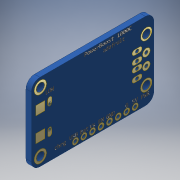
# Autodesk Inventor part: PlacaSuperboost1000C
Saved by Autodesk Inventor 2018 (Build 220112000, 112)
## iProperties
Created: 2018-01-30
Part Number: PlacaSuperboost1000C
Material: Genérico
Document SubType Name: Modeling
Designer: RafaX
Density: 1 g/cm^3
Appearance: Valor por defecto
Author: RafaX
Autodesk Inventor part; units mm, degrees
(part 1 of 2)
ref_plane "YZ Plane" through (0, 0, 0) normal (1, 0, 0) x (0, 1, 0)
ref_plane "XZ Plane" through (0, 0, 0) normal (0, 1, 0) x (-1, 0, 0)
ref_plane "PlanoCurre" through (0, 0, 0) normal (0, -1, 0) x (1, 0, 0)
sketch "FOTO_PLANO" plane through (0, 0, 0) normal (0, -1, 0) x (1, 0, 0)
  line L0 (-28.5613, 4.3764) -> (30.0496, 4.3764)
  line L1 (30.0496, 4.3764) -> (30.0496, -40.7266)
  line L2 (30.0496, -40.7266) -> (-28.5613, -40.7266)
  line L3 (-28.5613, -40.7266) -> (-28.5613, 4.3764)
  point P0 (0, 0)
  constraints: 2 other
sketch "BocetoPCB" plane through (0, 0, 0) normal (0, -1, 0) x (1, 0, 0)
  line L0 (-20.36, 0) -> (-2.5, 0)
  line L1 (0, -2.5) -> (0, -33.7)
  line L2 (-2.5, -36.2) -> (-20.36, -36.2)
  line L3 (-22.86, -33.7) -> (-22.86, -2.5)
  arc A0 (-20.36, 0) -> (-22.86, -2.5) centre (-20.36, -2.5) ccw
  arc A1 (0, -2.5) -> (-2.5, 0) centre (-2.5, -2.5) ccw
  arc A2 (-2.5, -36.2) -> (0, -33.7) centre (-2.5, -33.7) ccw
  arc A3 (-22.86, -33.7) -> (-20.36, -36.2) centre (-20.36, -33.7) ccw
  point P0 (-22.86, 0)
  point P1 (0, -36.2)
  point P2 (0, 0)
  point P3 (-20.255, -2.6419)
  point P4 (-2.605, -2.6419)
  point P5 (-0.0135, -33.9591)
  point P6 (-18.2509, -33.9512)
  point P7 (-5.1628, -33.9437)
  constraints: 9 point on circle, 8 end point, 8 tangent, 6 point on line, 4 centre point, 2 equal radius, 2 parallel, 1 horizontal, 1 perpendicular
extrude "board" add sketch "BocetoPCB" along normal blind 1.588
hole "Agujeros" at (-20.255, 0, -2.6419) at (-2.605, 0, -2.6419) at (-18.2509, 0, -33.9512) at (-5.1628, 0, -33.9437) direction (0, -1, 0) diameter 2.4 end through all
sketch "Boceto4" plane through (0, 0, 0) normal (0, 1, 0) x (1, 0, 0)
  circle A0 centre (-2.6033, 2.6414) radius 1.7995
  circle A1 centre (-2.6033, 2.6414) radius 1.2026
  circle A2 centre (-20.2425, 2.6414) radius 1.2088
  circle A3 centre (-20.2425, 2.6414) radius 1.8114
  circle A4 centre (-1.259, 13.0031) radius 0.4663
  circle A5 centre (-1.259, 13.0031) radius 0.9026
  circle A6 centre (-1.259, 15.5106) radius 0.4663
  circle A7 centre (-1.259, 15.5106) radius 0.9026
  circle A8 centre (-1.259, 18.0275) radius 0.4663
  circle A9 centre (-1.259, 18.0275) radius 0.9026
  circle A10 centre (-1.259, 20.5673) radius 0.4663
  circle A11 centre (-1.259, 20.5673) radius 0.9026
  circle A12 centre (-1.259, 23.0791) radius 0.4663
  circle A13 centre (-1.259, 23.0791) radius 0.9026
  circle A14 centre (-1.259, 25.6387) radius 0.4663
  circle A15 centre (-1.259, 25.6387) radius 0.9026
  circle A16 centre (-1.259, 28.1385) radius 0.4663
  circle A17 centre (-1.259, 28.1385) radius 0.9026
  circle A18 centre (-1.259, 30.6623) radius 0.4663
  circle A19 centre (-1.259, 30.6623) radius 0.9026
  circle A20 centre (-18.2509, 33.9512) radius 1.2 projected
  circle A21 centre (-18.2509, 33.9512) radius 1.2
  circle A22 centre (-18.2509, 33.9512) radius 1.6562
  circle A23 centre (-5.1628, 33.9437) radius 1.2 projected
  circle A24 centre (-5.1628, 33.9437) radius 1.2
  circle A25 centre (-5.1628, 33.9437) radius 1.6796
  circle A26 centre (-8.2006, 31.2204) radius 0.476
  line L0 (-8.2006, 29.7597) -> (-8.2006, 32.6808) construction
  line L1 (-7.4792, 30.4811) -> (-7.4792, 31.9594)
  line L2 (-8.9221, 31.9594) -> (-8.9221, 30.4811)
  arc A27 (-8.9221, 30.4811) -> (-7.4792, 30.4811) centre (-8.2006, 30.4811) ccw
  arc A28 (-7.4792, 31.9594) -> (-8.9221, 31.9594) centre (-8.2006, 31.9594) ccw
  circle A29 centre (-10.7403, 31.2204) radius 0.476
  line L3 (-10.0189, 30.4811) -> (-10.0189, 31.9594)
  line L4 (-11.4617, 31.9594) -> (-11.4617, 30.4811)
  arc A30 (-11.4617, 30.4811) -> (-10.0189, 30.4811) centre (-10.7403, 30.4811) ccw
  arc A31 (-10.0189, 31.9594) -> (-11.4617, 31.9594) centre (-10.7403, 31.9594) ccw
  circle A32 centre (-12.6758, 31.2204) radius 0.476
  line L5 (-11.9544, 30.4811) -> (-11.9544, 31.9594)
  line L6 (-13.3972, 31.9594) -> (-13.3972, 30.4811)
  arc A33 (-13.3972, 30.4811) -> (-11.9544, 30.4811) centre (-12.6758, 30.4811) ccw
  arc A34 (-11.9544, 31.9594) -> (-13.3972, 31.9594) centre (-12.6758, 31.9594) ccw
  circle A35 centre (-15.2037, 31.2204) radius 0.476
  line L7 (-14.4823, 30.4811) -> (-14.4823, 31.9594)
  line L8 (-15.9251, 31.9594) -> (-15.9251, 30.4811)
  arc A36 (-15.9251, 30.4811) -> (-14.4823, 30.4811) centre (-15.2037, 30.4811) ccw
  arc A37 (-14.4823, 31.9594) -> (-15.9251, 31.9594) centre (-15.2037, 31.9594) ccw
  line L9 (-16.2221, 1.3283) -> (-13.5843, 1.3283)
  line L10 (-13.5843, 1.3283) -> (-13.5843, 3.9523)
  line L11 (-13.5843, 3.9523) -> (-16.2221, 3.9523)
  line L12 (-16.2221, 3.9523) -> (-16.2221, 1.3283)
  line L13 (-9.0492, 1.3283) -> (-6.4567, 1.3283)
  line L14 (-6.4567, 1.3283) -> (-6.4567, 3.9523)
  line L15 (-6.4567, 3.9523) -> (-9.0492, 3.9523)
  line L16 (-9.0492, 3.9523) -> (-9.0492, 1.3283)
  line L17 (-16.4659, 5.4151) -> (-14.0753, 5.4151) construction
  line L18 (-15.8504, 4.7996) -> (-14.6908, 4.7996)
  line L19 (-14.6908, 6.0305) -> (-15.8504, 6.0305)
  arc A38 (-15.8504, 6.0305) -> (-15.8504, 4.7996) centre (-15.8504, 5.4151) ccw
  arc A39 (-14.6908, 4.7996) -> (-14.6908, 6.0305) centre (-14.6908, 5.4151) ccw
  circle A40 centre (-14.6284, 5.4151) radius 0.2973
  line L20 (-8.7027, 5.4177) -> (-6.2957, 5.4177) construction
  line L21 (-8.1043, 4.8193) -> (-6.8941, 4.8193)
  line L22 (-6.8941, 6.0161) -> (-8.1043, 6.0161)
  arc A41 (-8.1043, 6.0161) -> (-8.1043, 4.8193) centre (-8.1043, 5.4177) ccw
  arc A42 (-6.8941, 4.8193) -> (-6.8941, 6.0161) centre (-6.8941, 5.4177) ccw
  circle A43 centre (-8.1673, 5.4177) radius 0.2995
  circle A44 centre (-3.4049, 35.326) radius 0.1393
  circle A45 centre (-3.4049, 35.326) radius 0.4359
  circle A46 centre (-10.0649, 33.9437) radius 0.4442
  circle A47 centre (-10.0649, 33.9437) radius 1.1154
  circle A48 centre (-13.5064, 33.9548) radius 0.4442
  circle A49 centre (-13.5064, 33.9548) radius 1.1154
  line L23 (0, 33.7) -> (0, 2.5) projected
  circle A50 centre (-18.2509, 33.9512) radius 1.2 projected
  circle A51 centre (-20.255, 2.6419) radius 1.2 projected
  circle A52 centre (-2.605, 2.6419) radius 1.2 projected
  circle A53 centre (-5.1628, 33.9437) radius 1.2 projected
  line L24 (0, 2.5) -> (0, 33.7) projected
  arc A54 (0, 33.7) -> (-2.5, 36.2) centre (-2.5, 33.7) ccw projected
  line L25 (-2.5, 36.2) -> (-20.36, 36.2) projected
  arc A55 (-20.36, 36.2) -> (-22.86, 33.7) centre (-20.36, 33.7) ccw projected
  line L26 (-22.86, 33.7) -> (-22.86, 2.5) projected
  arc A56 (-22.86, 2.5) -> (-20.36, 0) centre (-20.36, 2.5) ccw projected
  line L27 (-20.36, 0) -> (-2.5, 0) projected
  arc A57 (-2.5, 0) -> (0, 2.5) centre (-2.5, 2.5) ccw projected
  point P0 (0, 0)
  point P1 (-8.2006, 31.2203)
  point P2 (-15.2706, 5.4151)
  point P3 (-7.4992, 5.4177)
  point P4 (-8.2006, 31.2203)
  constraints: 52 end point, 48 centre point, 30 point on circle, 24 tangent, 18 coincident, 10 parallel, 10 point on line, 4 horizontal, 3 midpoint, 2 perpendicular, 1 vertical
extrude "Extrusión3" add sketch "Boceto4" along normal blind 0.02 separate body contours A0 | A3 | A5 | A7 | A9 | A11 | A13 | A15 | A17 | A19 | A22 | A25 | A27 L2 A28 L1 | A30 L4 A31 L3 | A33 L6 A34 L5 | A36 L8 A37 L7 | L12 L11 L10 L9 | L16 L15 L14 L13 | A38 L19 A39 L18 | A41 L22 A42 L21 | A47 | A49
hole "Agujero4" at (-13.5064, 0, -33.9548) direction (0, -1, 0) diameter 1 end through all bodies 1
hole "Agujero5" at (-13.5064, 0, -33.9548) at (-10.0649, 0, -33.9437) at (-10.7403, 0, -31.2204) at (-12.6758, 0, -31.2204) at (-15.2037, 0, -31.2204) at (-8.2006, 0, -31.2203) at (-1.259, 0, -25.6387) at (-1.259, 0, -28.1385) at (-1.259, 0, -30.6623) at (-1.259, 0, -23.0791) at (-1.259, 0, -20.5673) at (-1.259, 0, -18.0275) at (-1.259, 0, -15.5106) at (-1.259, 0, -13.0031) at (-8.1673, 0, -5.4177) at (-14.6284, 0, -5.4151) direction (0, -1, 0) diameter 1 end through all bodies 1
sketch "textos" plane through (0, 0, 0) normal (0, 1, 0) x (1, 0, 0)
  line L0 (-22.5433, 15.6124) -> (-22.5433, 35.6124) construction
  line L1 (-22.5433, 35.6124) -> (-20.8728, 35.6124) construction
  line L2 (-20.8728, 35.6124) -> (-20.8728, 15.6124) construction
  line L3 (-20.8728, 15.6124) -> (-22.5433, 15.6124) construction
  line L4 (-20.9084, 21.173) -> (-20.9084, 28.7586) construction
  line L5 (-20.9084, 28.7586) -> (-19.6941, 28.7586) construction
  line L6 (-19.6941, 28.7586) -> (-19.6941, 21.173) construction
  line L7 (-19.6941, 21.173) -> (-20.9084, 21.173) construction
  line L8 (-3.3208, 11.209) -> (-3.3208, 13.795) construction
  line L9 (-3.3208, 13.795) -> (-2.293, 13.795) construction
  line L10 (-2.293, 13.795) -> (-2.293, 11.209) construction
  line L11 (-2.293, 11.209) -> (-3.3208, 11.209) construction
  line L12 (-3.274, 14.3294) -> (-3.274, 17.056) construction
  line L13 (-3.274, 17.056) -> (-2.274, 17.056) construction
  line L14 (-2.274, 17.056) -> (-2.274, 14.3294) construction
  line L15 (-2.274, 14.3294) -> (-3.274, 14.3294) construction
  line L16 (-3.2305, 17.2189) -> (-3.2305, 18.9429) construction
  line L17 (-3.2305, 18.9429) -> (-2.2171, 18.9429) construction
  line L18 (-2.2171, 18.9429) -> (-2.2171, 17.2189) construction
  line L19 (-2.2171, 17.2189) -> (-3.2305, 17.2189) construction
  line L20 (-3.274, 19.6989) -> (-3.274, 21.4229) construction
  line L21 (-3.274, 21.4229) -> (-2.274, 21.4229) construction
  line L22 (-2.274, 21.4229) -> (-2.274, 19.6989) construction
  line L23 (-2.274, 19.6989) -> (-3.274, 19.6989) construction
  line L24 (-3.3018, 22.0618) -> (-3.3018, 24.6478) construction
  line L25 (-3.3018, 24.6478) -> (-2.274, 24.6478) construction
  line L26 (-2.274, 24.6478) -> (-2.274, 22.0618) construction
  line L27 (-2.274, 22.0618) -> (-3.3018, 22.0618) construction
  line L28 (-3.3777, 27.7538) -> (-3.3777, 28.6158) construction
  line L29 (-3.3777, 28.6158) -> (-2.3499, 28.6158) construction
  line L30 (-2.3499, 28.6158) -> (-2.3499, 27.7538) construction
  line L31 (-2.3499, 27.7538) -> (-3.3777, 27.7538) construction
  line L32 (-3.3823, 29.7413) -> (-3.3823, 31.4654) construction
  line L33 (-3.3823, 31.4654) -> (-2.3689, 31.4654) construction
  line L34 (-2.3689, 31.4654) -> (-2.3689, 29.7413) construction
  line L35 (-2.3689, 29.7413) -> (-3.3823, 29.7413) construction
  line L36 (-3.255, 32.3541) -> (-3.255, 34.9402) construction
  line L37 (-3.255, 34.9402) -> (-2.255, 34.9402) construction
  line L38 (-2.255, 34.9402) -> (-2.255, 32.3541) construction
  line L39 (-2.255, 32.3541) -> (-3.255, 32.3541) construction
  line L40 (-3.0732, 6.7716) -> (-3.0732, 10.2196) construction
  line L41 (-3.0732, 10.2196) -> (-1.6699, 10.2196) construction
  line L42 (-1.6699, 10.2196) -> (-1.6699, 6.7716) construction
  line L43 (-1.6699, 6.7716) -> (-3.0732, 6.7716) construction
  line L44 (-18.5708, 4.0743) -> (-18.5708, 6.6604) construction
  line L45 (-18.5708, 6.6604) -> (-17.5431, 6.6604) construction
  line L46 (-17.5431, 6.6604) -> (-17.5431, 4.0743) construction
  line L47 (-17.5431, 4.0743) -> (-18.5708, 4.0743) construction
  line L48 (-17.5565, 4.8279) -> (-17.5565, 4.2527)
  line L49 (-17.5565, 4.2527) -> (-18.5565, 4.2527)
  line L50 (-18.5565, 4.2527) -> (-18.5565, 4.3915)
  line L51 (-18.5565, 4.3915) -> (-17.673, 4.3915)
  line L52 (-17.673, 4.3915) -> (-17.673, 4.8279)
  line L53 (-17.673, 4.8279) -> (-17.5565, 4.8279)
  spline S0 degree 2 poles (-18.0637, 5.7562) (-17.9284, 5.7562) (-17.733, 5.6926) (-17.6049, 5.5851) (-17.5431, 5.4399) (-17.5431, 5.3602) knots 0 0 0 1 2 3 4 4 4
  spline S1 degree 2 poles (-17.5431, 5.3602) (-17.5431, 5.2634) (-17.613, 5.12) (-17.7447, 5.026) (-17.9337, 4.9803) (-18.052, 4.9803) knots 0 0 0 1 2 3 4 4 4
  spline S2 degree 2 poles (-18.052, 4.9803) (-18.1855, 4.9803) (-18.3809, 5.043) (-18.509, 5.1505) (-18.5708, 5.2948) (-18.5708, 5.3754) knots 0 0 0 1 2 3 4 4 4
  spline S3 degree 2 poles (-18.5708, 5.3754) (-18.5708, 5.4713) (-18.5001, 5.6147) (-18.3692, 5.7096) (-18.1811, 5.7562) (-18.0637, 5.7562) knots 0 0 0 1 2 3 4 4 4
  spline S4 degree 2 poles (-18.0538, 5.62) (-18.1416, 5.62) (-18.2877, 5.5923) (-18.3934, 5.5313) (-18.4517, 5.4355) (-18.4517, 5.3674) knots 0 0 0 1 2 3 4 4 4
  spline S5 degree 2 poles (-18.4517, 5.3674) (-18.4517, 5.3019) (-18.3898, 5.207) (-18.2832, 5.146) (-18.1398, 5.1165) (-18.0592, 5.1165) knots 0 0 0 1 2 3 4 4 4
  spline S6 degree 2 poles (-18.0592, 5.1165) (-17.9705, 5.1165) (-17.8244, 5.1442) (-17.7196, 5.2052) (-17.6613, 5.3002) (-17.6613, 5.3674) knots 0 0 0 1 2 3 4 4 4
  spline S7 degree 2 poles (-17.6613, 5.3674) (-17.6613, 5.4328) (-17.7232, 5.5286) (-17.8298, 5.5905) (-17.9723, 5.62) (-18.0538, 5.62) knots 0 0 0 1 2 3 4 4 4
  line L54 (-18.5565, 6.6254) -> (-17.5565, 6.5582)
  line L55 (-17.5565, 6.5582) -> (-17.5565, 6.3817)
  line L56 (-17.5565, 6.3817) -> (-17.9122, 6.2571)
  line L57 (-17.9122, 6.2571) -> (-18.026, 6.2231)
  line L58 (-18.026, 6.2231) -> (-17.9033, 6.1872)
  line L59 (-17.9033, 6.1872) -> (-17.5565, 6.0717)
  line L60 (-17.5565, 6.0717) -> (-17.5565, 5.9014)
  line L61 (-17.5565, 5.9014) -> (-18.5565, 5.8324)
  line L62 (-18.5565, 5.8324) -> (-18.5565, 5.9605)
  line L63 (-18.5565, 5.9605) -> (-17.8755, 6)
  line L64 (-17.8755, 6) -> (-17.6891, 6.0116)
  line L65 (-17.6891, 6.0116) -> (-17.8477, 6.06)
  line L66 (-17.8477, 6.06) -> (-18.2187, 6.181)
  line L67 (-18.2187, 6.181) -> (-18.2187, 6.2751)
  line L68 (-18.2187, 6.2751) -> (-17.8208, 6.4148)
  line L69 (-17.8208, 6.4148) -> (-17.6891, 6.4614)
  line L70 (-17.6891, 6.4614) -> (-17.8262, 6.4641)
  line L71 (-17.8262, 6.4641) -> (-18.5565, 6.5036)
  line L72 (-18.5565, 6.5036) -> (-18.5565, 6.6254)
  line L73 (-19.8179, 21.7456) -> (-19.9209, 21.7429)
  spline S8 degree 2 poles (-19.9209, 21.7429) (-19.8591, 21.6846) (-19.8045, 21.5646) (-19.8045, 21.4983) knots 0 0 0 1 2 2 2
  spline S9 degree 2 poles (-19.8045, 21.4983) (-19.8045, 21.4373) (-19.8376, 21.3504) (-19.8968, 21.294) (-19.9765, 21.268) (-20.0231, 21.268) knots 0 0 0 1 2 3 4 4 4
  spline S10 degree 2 poles (-20.0231, 21.268) (-20.1387, 21.268) (-20.2695, 21.4275) (-20.2695, 21.5843) knots 0 0 0 1 2 2 2
  line L74 (-20.2695, 21.5843) -> (-20.2695, 21.7321)
  line L75 (-20.2695, 21.7321) -> (-20.3367, 21.7321)
  spline S11 degree 2 poles (-20.3367, 21.7321) (-20.4048, 21.7321) (-20.4864, 21.6515) (-20.4864, 21.5681) knots 0 0 0 1 2 2 2
  spline S12 degree 2 poles (-20.4864, 21.5681) (-20.4864, 21.5072) (-20.4577, 21.3898) (-20.4308, 21.3271) knots 0 0 0 1 2 2 2
  line L76 (-20.4308, 21.3271) -> (-20.5509, 21.3271)
  spline S13 degree 2 poles (-20.5509, 21.3271) (-20.5598, 21.3504) (-20.5778, 21.4086) (-20.5912, 21.4723) (-20.6002, 21.5422) (-20.6002, 21.578) knots 0 0 0 1 2 3 4 4 4
  spline S14 degree 2 poles (-20.6002, 21.578) (-20.6002, 21.6425) (-20.5697, 21.7465) (-20.507, 21.8181) (-20.412, 21.8567) (-20.3475, 21.8567) knots 0 0 0 1 2 3 4 4 4
  line L77 (-20.3475, 21.8567) -> (-19.8179, 21.8567)
  line L78 (-19.8179, 21.8567) -> (-19.8179, 21.7456)
  line L79 (-20.1674, 21.7321) -> (-20.1674, 21.5753)
  spline S15 degree 2 poles (-20.1674, 21.5753) (-20.1674, 21.5287) (-20.1476, 21.4615) (-20.1109, 21.4194) (-20.0598, 21.3988) (-20.0276, 21.3988) knots 0 0 0 1 2 3 4 4 4
  spline S16 degree 2 poles (-20.0276, 21.3988) (-20.0052, 21.3988) (-19.9649, 21.4113) (-19.9335, 21.44) (-19.9147, 21.4857) (-19.9147, 21.518) knots 0 0 0 1 2 3 4 4 4
  spline S17 degree 2 poles (-19.9147, 21.518) (-19.9147, 21.561) (-19.9711, 21.6712) (-20.0312, 21.7321) knots 0 0 0 1 2 2 2
  line L80 (-20.0312, 21.7321) -> (-20.1674, 21.7321)
  spline S18 degree 2 poles (-20.1862, 22.052) (-20.2838, 22.052) (-20.4362, 22.1013) (-20.541, 22.1936) (-20.5957, 22.3217) (-20.5957, 22.4006) knots 0 0 0 1 2 3 4 4 4
  spline S19 degree 2 poles (-20.5957, 22.4006) (-20.5957, 22.4346) (-20.5858, 22.5009) (-20.576, 22.5332) knots 0 0 0 1 2 2 2
  line L81 (-20.576, 22.5332) -> (-20.8994, 22.5332)
  line L82 (-20.8994, 22.5332) -> (-20.8994, 22.6577)
  line L83 (-20.8994, 22.6577) -> (-19.8179, 22.6577)
  line L84 (-19.8179, 22.6577) -> (-19.8179, 22.5466)
  line L85 (-19.8179, 22.5466) -> (-19.9631, 22.5422)
  spline S20 degree 2 poles (-19.9631, 22.5422) (-19.8824, 22.4902) (-19.8045, 22.3692) (-19.8045, 22.2993) knots 0 0 0 1 2 2 2
  spline S21 degree 2 poles (-19.8045, 22.2993) (-19.8045, 22.2384) (-19.8591, 22.1452) (-19.9595, 22.0825) (-20.1002, 22.052) (-20.1862, 22.052) knots 0 0 0 1 2 3 4 4 4
  spline S22 degree 2 poles (-20.1942, 22.1784) (-20.0554, 22.1784) (-19.9183, 22.2545) (-19.9183, 22.3244) knots 0 0 0 1 2 2 2
  spline S23 degree 2 poles (-19.9183, 22.3244) (-19.9183, 22.371) (-20.0088, 22.4758) (-20.0975, 22.5332) knots 0 0 0 1 2 2 2
  line L86 (-20.0975, 22.5332) -> (-20.4541, 22.5332)
  spline S24 degree 2 poles (-20.4541, 22.5332) (-20.4693, 22.5027) (-20.4855, 22.4284) (-20.4855, 22.3925) knots 0 0 0 1 2 2 2
  spline S25 degree 2 poles (-20.4855, 22.3925) (-20.4855, 22.2913) (-20.3448, 22.1784) (-20.1942, 22.1784) knots 0 0 0 1 2 2 2
  line L87 (-19.8179, 23.3477) -> (-19.9209, 23.345)
  spline S26 degree 2 poles (-19.9209, 23.345) (-19.8591, 23.2868) (-19.8045, 23.1667) (-19.8045, 23.1004) knots 0 0 0 1 2 2 2
  spline S27 degree 2 poles (-19.8045, 23.1004) (-19.8045, 23.0395) (-19.8376, 22.9526) (-19.8968, 22.8961) (-19.9765, 22.8701) (-20.0231, 22.8701) knots 0 0 0 1 2 3 4 4 4
  spline S28 degree 2 poles (-20.0231, 22.8701) (-20.1387, 22.8701) (-20.2695, 23.0296) (-20.2695, 23.1864) knots 0 0 0 1 2 2 2
  line L88 (-20.2695, 23.1864) -> (-20.2695, 23.3343)
  line L89 (-20.2695, 23.3343) -> (-20.3367, 23.3343)
  spline S29 degree 2 poles (-20.3367, 23.3343) (-20.4048, 23.3343) (-20.4864, 23.2536) (-20.4864, 23.1703) knots 0 0 0 1 2 2 2
  spline S30 degree 2 poles (-20.4864, 23.1703) (-20.4864, 23.1094) (-20.4577, 22.992) (-20.4308, 22.9293) knots 0 0 0 1 2 2 2
  line L90 (-20.4308, 22.9293) -> (-20.5509, 22.9293)
  spline S31 degree 2 poles (-20.5509, 22.9293) (-20.5598, 22.9526) (-20.5778, 23.0108) (-20.5912, 23.0744) (-20.6002, 23.1443) (-20.6002, 23.1802) knots 0 0 0 1 2 3 4 4 4
  spline S32 degree 2 poles (-20.6002, 23.1802) (-20.6002, 23.2447) (-20.5697, 23.3486) (-20.507, 23.4203) (-20.412, 23.4588) (-20.3475, 23.4588) knots 0 0 0 1 2 3 4 4 4
  line L91 (-20.3475, 23.4588) -> (-19.8179, 23.4588)
  line L92 (-19.8179, 23.4588) -> (-19.8179, 23.3477)
  line L93 (-20.1674, 23.3343) -> (-20.1674, 23.1775)
  spline S33 degree 2 poles (-20.1674, 23.1775) (-20.1674, 23.1309) (-20.1476, 23.0637) (-20.1109, 23.0215) (-20.0598, 23.0009) (-20.0276, 23.0009) knots 0 0 0 1 2 3 4 4 4
  spline S34 degree 2 poles (-20.0276, 23.0009) (-20.0052, 23.0009) (-19.9649, 23.0135) (-19.9335, 23.0422) (-19.9147, 23.0879) (-19.9147, 23.1201) knots 0 0 0 1 2 3 4 4 4
  spline S35 degree 2 poles (-19.9147, 23.1201) (-19.9147, 23.1631) (-19.9711, 23.2733) (-20.0312, 23.3343) knots 0 0 0 1 2 2 2
  line L94 (-20.0312, 23.3343) -> (-20.1674, 23.3343)
  spline S36 degree 2 poles (-20.7749, 24.3235) (-20.7973, 24.2267) (-20.7973, 24.156) knots 0 0 0 1 1 1
  spline S37 degree 2 poles (-20.7973, 24.156) (-20.7973, 23.9884) (-20.6091, 23.9884) knots 0 0 0 1 1 1
  line L95 (-20.6091, 23.9884) -> (-20.4747, 23.9884)
  line L96 (-20.4747, 23.9884) -> (-20.4747, 24.302)
  line L97 (-20.4747, 24.302) -> (-20.3636, 24.302)
  line L98 (-20.3636, 24.302) -> (-20.3636, 23.9884)
  line L99 (-20.3636, 23.9884) -> (-19.8179, 23.9884)
  line L100 (-19.8179, 23.9884) -> (-19.8179, 23.8629)
  line L101 (-19.8179, 23.8629) -> (-20.3636, 23.8629)
  line L102 (-20.3636, 23.8629) -> (-20.3636, 23.6336)
  line L103 (-20.3636, 23.6336) -> (-20.4747, 23.6336)
  line L104 (-20.4747, 23.6336) -> (-20.4747, 23.8629)
  line L105 (-20.4747, 23.8629) -> (-20.602, 23.8629)
  spline S38 degree 2 poles (-20.602, 23.8629) (-20.9084, 23.8629) (-20.9084, 24.1604) knots 0 0 0 1 1 1
  spline S39 degree 2 poles (-20.9084, 24.1604) (-20.9084, 24.2339) (-20.8896, 24.3235) knots 0 0 0 1 1 1
  line L106 (-20.8896, 24.3235) -> (-20.7749, 24.3235)
  line L107 (-20.5858, 24.5207) -> (-20.5858, 24.6336)
  line L108 (-20.5858, 24.6336) -> (-20.4442, 24.6371)
  spline S40 degree 2 poles (-20.4442, 24.6371) (-20.5267, 24.6999) (-20.6002, 24.8235) (-20.6002, 24.8862) knots 0 0 0 1 2 2 2
  spline S41 degree 2 poles (-20.6002, 24.8862) (-20.6002, 24.9974) (-20.4451, 25.1112) (-20.2928, 25.1076) knots 0 0 0 1 2 2 2
  line L109 (-20.2928, 25.1076) -> (-20.2928, 24.9821)
  spline S42 degree 2 poles (-20.2928, 24.9821) (-20.3941, 24.9839) (-20.4855, 24.9248) (-20.4855, 24.8683) knots 0 0 0 1 2 2 2
  spline S43 degree 2 poles (-20.4855, 24.8683) (-20.4855, 24.8432) (-20.4657, 24.7931) (-20.4236, 24.7393) (-20.3582, 24.6793) (-20.3116, 24.6452) knots 0 0 0 1 2 3 4 4 4
  line L110 (-20.3116, 24.6452) -> (-19.8179, 24.6452)
  line L111 (-19.8179, 24.6452) -> (-19.8179, 24.5207)
  line L112 (-19.8179, 24.5207) -> (-20.5858, 24.5207)
  line L113 (-19.8179, 25.8665) -> (-19.8179, 25.7554)
  line L114 (-19.8179, 25.7554) -> (-19.9416, 25.7509)
  spline S44 degree 2 poles (-19.9416, 25.7509) (-19.9021, 25.7187) (-19.8493, 25.6613) (-19.817, 25.6049) (-19.8045, 25.5466) (-19.8045, 25.5153) knots 0 0 0 1 2 3 4 4 4
  spline S45 degree 2 poles (-19.8045, 25.5153) (-19.8045, 25.4042) (-19.9433, 25.2922) (-20.084, 25.2922) knots 0 0 0 1 2 2 2
  line L115 (-20.084, 25.2922) -> (-20.5858, 25.2922)
  line L116 (-20.5858, 25.2922) -> (-20.5858, 25.4158)
  line L117 (-20.5858, 25.4158) -> (-20.0948, 25.4158)
  spline S46 degree 2 poles (-20.0948, 25.4158) (-19.9183, 25.4158) (-19.9183, 25.5395) knots 0 0 0 1 1 1
  spline S47 degree 2 poles (-19.9183, 25.5395) (-19.9183, 25.5628) (-19.9326, 25.6058) (-19.9684, 25.6533) (-20.0303, 25.7079) (-20.0769, 25.7429) knots 0 0 0 1 2 3 4 4 4
  line L118 (-20.0769, 25.7429) -> (-20.5858, 25.7429)
  line L119 (-20.5858, 25.7429) -> (-20.5858, 25.8665)
  line L120 (-20.5858, 25.8665) -> (-19.8179, 25.8665)
  line L121 (-20.4756, 26.337) -> (-20.4756, 26.1255)
  line L122 (-20.4756, 26.1255) -> (-20.5858, 26.1255)
  line L123 (-20.5858, 26.1255) -> (-20.5858, 26.4615)
  line L124 (-20.5858, 26.4615) -> (-19.929, 26.4615)
  line L125 (-19.929, 26.4615) -> (-19.929, 26.6748)
  line L126 (-19.929, 26.6748) -> (-19.8179, 26.6748)
  line L127 (-19.8179, 26.6748) -> (-19.8179, 26.1022)
  line L128 (-19.8179, 26.1022) -> (-19.929, 26.1022)
  line L129 (-19.929, 26.1022) -> (-19.929, 26.337)
  line L130 (-19.929, 26.337) -> (-20.4756, 26.337)
  spline S48 degree 2 poles (-20.9084, 26.38) (-20.9084, 26.4006) (-20.8923, 26.4364) (-20.8636, 26.4624) (-20.826, 26.4776) (-20.8036, 26.4776) knots 0 0 0 1 2 3 4 4 4
  spline S49 degree 2 poles (-20.8036, 26.4776) (-20.7821, 26.4776) (-20.7435, 26.4624) (-20.7149, 26.4364) (-20.6987, 26.4006) (-20.6987, 26.38) knots 0 0 0 1 2 3 4 4 4
  spline S50 degree 2 poles (-20.6987, 26.38) (-20.6987, 26.3594) (-20.7149, 26.3235) (-20.7435, 26.2975) (-20.7821, 26.2823) (-20.8036, 26.2823) knots 0 0 0 1 2 3 4 4 4
  spline S51 degree 2 poles (-20.8036, 26.2823) (-20.826, 26.2823) (-20.8636, 26.2975) (-20.8923, 26.3235) (-20.9084, 26.3594) (-20.9084, 26.38) knots 0 0 0 1 2 3 4 4 4
  spline S52 degree 2 poles (-19.8287, 27.4696) (-19.817, 27.4275) (-19.8071, 27.3379) (-19.8071, 27.2922) knots 0 0 0 1 2 2 2
  spline S53 degree 2 poles (-19.8071, 27.2922) (-19.8071, 27.1577) (-19.938, 27.0251) (-20.0733, 27.0251) knots 0 0 0 1 2 2 2
  line L131 (-20.0733, 27.0251) -> (-20.4747, 27.0251)
  line L132 (-20.4747, 27.0251) -> (-20.4747, 26.8253)
  line L133 (-20.4747, 26.8253) -> (-20.5858, 26.8253)
  line L134 (-20.5858, 26.8253) -> (-20.5858, 27.0251)
  line L135 (-20.5858, 27.0251) -> (-20.7973, 27.0251)
  line L136 (-20.7973, 27.0251) -> (-20.8322, 27.1488)
  line L137 (-20.8322, 27.1488) -> (-20.5858, 27.1488)
  line L138 (-20.5858, 27.1488) -> (-20.5858, 27.4696)
  line L139 (-20.5858, 27.4696) -> (-20.4747, 27.4696)
  line L140 (-20.4747, 27.4696) -> (-20.4747, 27.1488)
  line L141 (-20.4747, 27.1488) -> (-20.084, 27.1488)
  spline S54 degree 2 poles (-20.084, 27.1488) (-20.0016, 27.1488) (-19.9201, 27.2312) (-19.9201, 27.3101) knots 0 0 0 1 2 2 2
  spline S55 degree 2 poles (-19.9201, 27.3101) (-19.9201, 27.345) (-19.9308, 27.4257) (-19.9433, 27.4696) knots 0 0 0 1 2 2 2
  line L142 (-19.9433, 27.4696) -> (-19.8287, 27.4696)
  spline S56 degree 2 poles (-22.1992, 16.426) (-22.1212, 16.426) (-21.9886, 16.3722) (-21.8918, 16.2683) (-21.839, 16.1124) (-21.839, 16.0093) knots 0 0 0 1 2 3 4 4 4
  line L143 (-21.839, 16.0093) -> (-21.839, 15.9117)
  line L144 (-21.839, 15.9117) -> (-21.5173, 15.9117)
  line L145 (-21.5173, 15.9117) -> (-21.5173, 15.7181)
  line L146 (-21.5173, 15.7181) -> (-22.5173, 15.7181)
  line L147 (-22.5173, 15.7181) -> (-22.5173, 16.0165)
  spline S57 degree 2 poles (-22.5173, 16.0165) (-22.5173, 16.116) (-22.4752, 16.2683) (-22.3945, 16.3722) (-22.2754, 16.426) (-22.1992, 16.426) knots 0 0 0 1 2 3 4 4 4
  spline S58 degree 2 poles (-22.1857, 16.2244) (-22.2261, 16.2244) (-22.2906, 16.1984) (-22.3372, 16.1464) (-22.3614, 16.0667) (-22.3614, 16.012) knots 0 0 0 1 2 3 4 4 4
  line L148 (-22.3614, 16.012) -> (-22.3614, 15.9117)
  line L149 (-22.3614, 15.9117) -> (-21.9949, 15.9117)
  line L150 (-21.9949, 15.9117) -> (-21.9949, 16.0183)
  spline S59 degree 2 poles (-21.9949, 16.0183) (-21.9949, 16.0685) (-22.0218, 16.1446) (-22.0719, 16.1966) (-22.1427, 16.2244) (-22.1857, 16.2244) knots 0 0 0 1 2 3 4 4 4
  spline S60 degree 2 poles (-21.9124, 17.314) (-21.8202, 17.314) (-21.6678, 17.2611) (-21.5594, 17.1608) (-21.4994, 17.0156) (-21.4994, 16.9233) knots 0 0 0 1 2 3 4 4 4
  spline S61 degree 2 poles (-21.4994, 16.9233) (-21.4994, 16.8346) (-21.5504, 16.6957) (-21.6508, 16.5989) (-21.8013, 16.5479) (-21.9017, 16.5479) knots 0 0 0 1 2 3 4 4 4
  spline S62 degree 2 poles (-21.9017, 16.5479) (-21.994, 16.5479) (-22.1454, 16.6016) (-22.2529, 16.702) (-22.3112, 16.8471) (-22.3112, 16.9385) knots 0 0 0 1 2 3 4 4 4
  spline S63 degree 2 poles (-22.3112, 16.9385) (-22.3112, 17.0272) (-22.2601, 17.167) (-22.1598, 17.2638) (-22.0101, 17.314) (-21.9124, 17.314) knots 0 0 0 1 2 3 4 4 4
  spline S64 degree 2 poles (-21.908, 17.116) (-22.028, 17.116) (-22.1499, 17.0228) (-22.1499, 16.9323) knots 0 0 0 1 2 2 2
  spline S65 degree 2 poles (-22.1499, 16.9323) (-22.1499, 16.8821) (-22.1123, 16.8122) (-22.0451, 16.7674) (-21.9564, 16.7459) (-21.9062, 16.7459) knots 0 0 0 1 2 3 4 4 4
  spline S66 degree 2 poles (-21.9062, 16.7459) (-21.7843, 16.7459) (-21.6616, 16.8453) (-21.6616, 16.9323) knots 0 0 0 1 2 2 2
  spline S67 degree 2 poles (-21.6616, 16.9323) (-21.6616, 16.9798) (-21.6983, 17.0505) (-21.7655, 17.0936) (-21.8551, 17.116) (-21.908, 17.116) knots 0 0 0 1 2 3 4 4 4
  line L151 (-21.5173, 18.1303) -> (-21.5173, 17.9188)
  line L152 (-21.5173, 17.9188) -> (-21.7637, 17.8337)
  line L153 (-21.7637, 17.8337) -> (-21.8497, 17.8086)
  line L154 (-21.8497, 17.8086) -> (-21.761, 17.7826)
  line L155 (-21.761, 17.7826) -> (-21.5173, 17.7011)
  line L156 (-21.5173, 17.7011) -> (-21.5173, 17.4887)
  line L157 (-21.5173, 17.4887) -> (-22.2951, 17.3767)
  line L158 (-22.2951, 17.3767) -> (-22.2951, 17.5577)
  line L159 (-22.2951, 17.5577) -> (-21.8551, 17.6151)
  line L160 (-21.8551, 17.6151) -> (-21.735, 17.6276)
  line L161 (-21.735, 17.6276) -> (-21.8435, 17.6599)
  line L162 (-21.8435, 17.6599) -> (-22.08, 17.7396)
  line L163 (-22.08, 17.7396) -> (-22.08, 17.8848)
  line L164 (-22.08, 17.8848) -> (-21.8452, 17.9699)
  line L165 (-21.8452, 17.9699) -> (-21.7341, 18.0066)
  line L166 (-21.7341, 18.0066) -> (-21.8569, 18.0219)
  line L167 (-21.8569, 18.0219) -> (-22.2951, 18.0694)
  line L168 (-22.2951, 18.0694) -> (-22.2951, 18.2414)
  line L169 (-22.2951, 18.2414) -> (-21.5173, 18.1303)
  spline S68 degree 2 poles (-21.9653, 19.0488) (-21.9465, 19.0488) (-21.8856, 19.0461) (-21.8587, 19.0443) knots 0 0 0 1 2 2 2
  line L170 (-21.8587, 19.0443) -> (-21.8587, 18.5228)
  spline S69 degree 2 poles (-21.8587, 18.5228) (-21.8076, 18.5228) (-21.7297, 18.555) (-21.6768, 18.6133) (-21.649, 18.6948) (-21.649, 18.745) knots 0 0 0 1 2 3 4 4 4
  spline S70 degree 2 poles (-21.649, 18.745) (-21.649, 18.8032) (-21.6669, 18.935) (-21.6866, 19.0057) knots 0 0 0 1 2 2 2
  line L171 (-21.6866, 19.0057) -> (-21.5379, 19.0057)
  spline S71 degree 2 poles (-21.5379, 19.0057) (-21.5298, 18.9753) (-21.5155, 18.9036) (-21.5047, 18.8283) (-21.4994, 18.7522) (-21.4994, 18.7163) knots 0 0 0 1 2 3 4 4 4
  spline S72 degree 2 poles (-21.4994, 18.7163) (-21.4994, 18.6258) (-21.5504, 18.4824) (-21.649, 18.3821) (-21.7942, 18.3292) (-21.89, 18.3292) knots 0 0 0 1 2 3 4 4 4
  spline S73 degree 2 poles (-21.89, 18.3292) (-21.985, 18.3292) (-22.14, 18.3821) (-22.2512, 18.4789) (-22.3112, 18.6169) (-22.3112, 18.702) knots 0 0 0 1 2 3 4 4 4
  spline S74 degree 2 poles (-22.3112, 18.702) (-22.3112, 18.7862) (-22.2601, 18.9161) (-22.1687, 19.0031) (-22.0415, 19.0488) (-21.9653, 19.0488) knots 0 0 0 1 2 3 4 4 4
  spline S75 degree 2 poles (-21.9922, 18.8552) (-22.0388, 18.8561) (-22.1069, 18.831) (-22.1508, 18.788) (-22.1723, 18.7307) (-22.1723, 18.6984) knots 0 0 0 1 2 3 4 4 4
  spline S76 degree 2 poles (-22.1723, 18.6984) (-22.1723, 18.6267) (-22.0782, 18.5344) (-21.9922, 18.5255) knots 0 0 0 1 2 2 2
  line L172 (-21.9922, 18.5255) -> (-21.9922, 18.8552)
  spline S77 degree 2 poles (-21.9922, 19.7477) (-22.0361, 19.7495) (-22.097, 19.7369) (-22.1374, 19.7118) (-22.1553, 19.6742) (-22.1553, 19.65) knots 0 0 0 1 2 3 4 4 4
  spline S78 degree 2 poles (-22.1553, 19.65) (-22.1553, 19.6079) (-22.0872, 19.5183) (-22.0092, 19.4645) knots 0 0 0 1 2 2 2
  line L173 (-22.0092, 19.4645) -> (-21.5173, 19.4645)
  line L174 (-21.5173, 19.4645) -> (-21.5173, 19.2692)
  line L175 (-21.5173, 19.2692) -> (-22.2951, 19.2692)
  line L176 (-22.2951, 19.2692) -> (-22.2951, 19.4412)
  line L177 (-22.2951, 19.4412) -> (-22.1813, 19.4484)
  spline S79 degree 2 poles (-22.1813, 19.4484) (-22.2117, 19.4681) (-22.2592, 19.5174) (-22.2933, 19.5774) (-22.3112, 19.6509) (-22.3112, 19.6948) knots 0 0 0 1 2 3 4 4 4
  spline S80 degree 2 poles (-22.3112, 19.6948) (-22.3112, 19.7548) (-22.2709, 19.8471) (-22.1911, 19.9108) (-22.071, 19.9412) (-21.9922, 19.9385) knots 0 0 0 1 2 3 4 4 4
  line L178 (-21.9922, 19.9385) -> (-21.9922, 19.7477)
  line L179 (-21.5173, 20.1079) -> (-22.5173, 20.1079)
  line L180 (-22.5173, 20.1079) -> (-22.5173, 20.4376)
  spline S81 degree 2 poles (-22.5173, 20.4376) (-22.5173, 20.6115) (-22.3981, 20.7853) (-22.2771, 20.7853) knots 0 0 0 1 2 2 2
  spline S82 degree 2 poles (-22.2771, 20.7853) (-22.2395, 20.7853) (-22.1687, 20.7674) (-22.1087, 20.7307) (-22.063, 20.6742) (-22.0495, 20.6357) knots 0 0 0 1 2 3 4 4 4
  spline S83 degree 2 poles (-22.0495, 20.6357) (-22.0442, 20.6742) (-22.0074, 20.7432) (-21.9501, 20.7961) (-21.8721, 20.8265) (-21.8237, 20.8265) knots 0 0 0 1 2 3 4 4 4
  spline S84 degree 2 poles (-21.8237, 20.8265) (-21.6714, 20.8265) (-21.5173, 20.6169) (-21.5173, 20.4197) knots 0 0 0 1 2 2 2
  line L181 (-21.5173, 20.4197) -> (-21.5173, 20.1079)
  spline S85 degree 2 poles (-21.6714, 20.4332) (-21.6714, 20.4789) (-21.6938, 20.5488) (-21.735, 20.5953) (-21.7897, 20.6195) (-21.821, 20.6195) knots 0 0 0 1 2 3 4 4 4
  spline S86 degree 2 poles (-21.821, 20.6195) (-21.8865, 20.6195) (-21.9599, 20.5201) (-21.9599, 20.4179) knots 0 0 0 1 2 2 2
  line L182 (-21.9599, 20.4179) -> (-21.9599, 20.2988)
  line L183 (-21.9599, 20.2988) -> (-21.6714, 20.2988)
  line L184 (-21.6714, 20.2988) -> (-21.6714, 20.4332)
  spline S87 degree 2 poles (-22.244, 20.5855) (-22.2727, 20.5855) (-22.3184, 20.5676) (-22.3506, 20.5255) (-22.3685, 20.4609) (-22.3685, 20.4152) knots 0 0 0 1 2 3 4 4 4
  line L185 (-22.3685, 20.4152) -> (-22.3685, 20.2988)
  line L186 (-22.3685, 20.2988) -> (-22.1033, 20.2988)
  line L187 (-22.1033, 20.2988) -> (-22.1033, 20.4152)
  spline S88 degree 2 poles (-22.1033, 20.4152) (-22.1033, 20.4618) (-22.1257, 20.5264) (-22.1642, 20.5676) (-22.2153, 20.5855) (-22.244, 20.5855) knots 0 0 0 1 2 3 4 4 4
  spline S89 degree 2 poles (-21.9124, 21.7091) (-21.8202, 21.7091) (-21.6678, 21.6563) (-21.5594, 21.5559) (-21.4994, 21.4108) (-21.4994, 21.3185) knots 0 0 0 1 2 3 4 4 4
  spline S90 degree 2 poles (-21.4994, 21.3185) (-21.4994, 21.2298) (-21.5504, 21.0909) (-21.6508, 20.9941) (-21.8013, 20.943) (-21.9017, 20.943) knots 0 0 0 1 2 3 4 4 4
  spline S91 degree 2 poles (-21.9017, 20.943) (-21.994, 20.943) (-22.1454, 20.9968) (-22.2529, 21.0971) (-22.3112, 21.2423) (-22.3112, 21.3337) knots 0 0 0 1 2 3 4 4 4
  spline S92 degree 2 poles (-22.3112, 21.3337) (-22.3112, 21.4224) (-22.2601, 21.5622) (-22.1598, 21.659) (-22.0101, 21.7091) (-21.9124, 21.7091) knots 0 0 0 1 2 3 4 4 4
  spline S93 degree 2 poles (-21.908, 21.5111) (-22.028, 21.5111) (-22.1499, 21.4179) (-22.1499, 21.3274) knots 0 0 0 1 2 2 2
  spline S94 degree 2 poles (-22.1499, 21.3274) (-22.1499, 21.2772) (-22.1123, 21.2074) (-22.0451, 21.1626) (-21.9564, 21.141) (-21.9062, 21.141) knots 0 0 0 1 2 3 4 4 4
  spline S95 degree 2 poles (-21.9062, 21.141) (-21.7843, 21.141) (-21.6616, 21.2405) (-21.6616, 21.3274) knots 0 0 0 1 2 2 2
  spline S96 degree 2 poles (-21.6616, 21.3274) (-21.6616, 21.3749) (-21.6983, 21.4457) (-21.7655, 21.4887) (-21.8551, 21.5111) (-21.908, 21.5111) knots 0 0 0 1 2 3 4 4 4
  spline S97 degree 2 poles (-21.9124, 22.5882) (-21.8202, 22.5882) (-21.6678, 22.5353) (-21.5594, 22.435) (-21.4994, 22.2898) (-21.4994, 22.1975) knots 0 0 0 1 2 3 4 4 4
  spline S98 degree 2 poles (-21.4994, 22.1975) (-21.4994, 22.1088) (-21.5504, 21.9699) (-21.6508, 21.8731) (-21.8013, 21.8221) (-21.9017, 21.8221) knots 0 0 0 1 2 3 4 4 4
  spline S99 degree 2 poles (-21.9017, 21.8221) (-21.994, 21.8221) (-22.1454, 21.8758) (-22.2529, 21.9762) (-22.3112, 22.1213) (-22.3112, 22.2127) knots 0 0 0 1 2 3 4 4 4
  spline S100 degree 2 poles (-22.3112, 22.2127) (-22.3112, 22.3014) (-22.2601, 22.4412) (-22.1598, 22.538) (-22.0101, 22.5882) (-21.9124, 22.5882) knots 0 0 0 1 2 3 4 4 4
  spline S101 degree 2 poles (-21.908, 22.3902) (-22.028, 22.3902) (-22.1499, 22.297) (-22.1499, 22.2065) knots 0 0 0 1 2 2 2
  spline S102 degree 2 poles (-22.1499, 22.2065) (-22.1499, 22.1563) (-22.1123, 22.0864) (-22.0451, 22.0416) (-21.9564, 22.0201) (-21.9062, 22.0201) knots 0 0 0 1 2 3 4 4 4
  spline S103 degree 2 poles (-21.9062, 22.0201) (-21.7843, 22.0201) (-21.6616, 22.1195) (-21.6616, 22.2065) knots 0 0 0 1 2 2 2
  spline S104 degree 2 poles (-21.6616, 22.2065) (-21.6616, 22.2539) (-21.6983, 22.3247) (-21.7655, 22.3677) (-21.8551, 22.3902) (-21.908, 22.3902) knots 0 0 0 1 2 3 4 4 4
  spline S105 degree 2 poles (-21.7458, 23.4072) (-21.6795, 23.4072) (-21.5854, 23.3471) (-21.5262, 23.2477) (-21.4994, 23.1222) (-21.4994, 23.0568) knots 0 0 0 1 2 3 4 4 4
  spline S106 degree 2 poles (-21.4994, 23.0568) (-21.4994, 22.969) (-21.5155, 22.8292) (-21.5307, 22.7665) knots 0 0 0 1 2 2 2
  line L188 (-21.5307, 22.7665) -> (-21.6992, 22.7665)
  spline S107 degree 2 poles (-21.6992, 22.7665) (-21.6696, 22.84) (-21.6427, 22.986) (-21.6427, 23.0505) knots 0 0 0 1 2 2 2
  spline S108 degree 2 poles (-21.6427, 23.0505) (-21.6427, 23.1258) (-21.6893, 23.1993) (-21.727, 23.1993) knots 0 0 0 1 2 2 2
  spline S109 degree 2 poles (-21.727, 23.1993) (-21.7449, 23.1993) (-21.7736, 23.1841) (-21.8004, 23.141) (-21.8291, 23.0631) (-21.8461, 22.9995) knots 0 0 0 1 2 3 4 4 4
  spline S110 degree 2 poles (-21.8461, 22.9995) (-21.8623, 22.9412) (-21.9026, 22.8534) (-21.9581, 22.7952) (-22.0307, 22.7665) (-22.08, 22.7665) knots 0 0 0 1 2 3 4 4 4
  spline S111 degree 2 poles (-22.08, 22.7665) (-22.1275, 22.7665) (-22.2117, 22.8104) (-22.2745, 22.8964) (-22.3112, 23.0264) (-22.3112, 23.1133) knots 0 0 0 1 2 3 4 4 4
  spline S112 degree 2 poles (-22.3112, 23.1133) (-22.3112, 23.1876) (-22.296, 23.3032) (-22.287, 23.348) knots 0 0 0 1 2 2 2
  line L189 (-22.287, 23.348) -> (-22.1347, 23.348)
  spline S113 degree 2 poles (-22.1347, 23.348) (-22.1562, 23.2799) (-22.1741, 23.1608) (-22.1741, 23.1016) knots 0 0 0 1 2 2 2
  spline S114 degree 2 poles (-22.1741, 23.1016) (-22.1741, 23.0434) (-22.1329, 22.9726) (-22.0961, 22.9726) knots 0 0 0 1 2 2 2
  spline S115 degree 2 poles (-22.0961, 22.9726) (-22.0782, 22.9726) (-22.0504, 22.9869) (-22.0245, 23.0281) (-21.9967, 23.1016) (-21.9797, 23.1626) knots 0 0 0 1 2 3 4 4 4
  spline S116 degree 2 poles (-21.9797, 23.1626) (-21.9599, 23.2315) (-21.9169, 23.3256) (-21.8614, 23.3821) (-21.7915, 23.4072) (-21.7458, 23.4072) knots 0 0 0 1 2 3 4 4 4
  spline S117 degree 2 poles (-21.5254, 24.2862) (-21.5137, 24.2351) (-21.4994, 24.1303) (-21.4994, 24.0837) knots 0 0 0 1 2 2 2
  spline S118 degree 2 poles (-21.4994, 24.0837) (-21.4994, 24.0048) (-21.5316, 23.8919) (-21.5979, 23.8176) (-21.6992, 23.7826) (-21.77, 23.7826) knots 0 0 0 1 2 3 4 4 4
  line L190 (-21.77, 23.7826) -> (-22.149, 23.7826)
  line L191 (-22.149, 23.7826) -> (-22.149, 23.5694)
  line L192 (-22.149, 23.5694) -> (-22.2951, 23.5694)
  line L193 (-22.2951, 23.5694) -> (-22.2951, 23.7826)
  line L194 (-22.2951, 23.7826) -> (-22.494, 23.7826)
  line L195 (-22.494, 23.7826) -> (-22.5433, 23.978)
  line L196 (-22.5433, 23.978) -> (-22.2951, 23.978)
  line L197 (-22.2951, 23.978) -> (-22.2951, 24.2862)
  line L198 (-22.2951, 24.2862) -> (-22.149, 24.2862)
  line L199 (-22.149, 24.2862) -> (-22.149, 23.978)
  line L200 (-22.149, 23.978) -> (-21.7834, 23.978)
  spline S119 degree 2 poles (-21.7834, 23.978) (-21.7171, 23.978) (-21.649, 24.0407) (-21.649, 24.1142) knots 0 0 0 1 2 2 2
  spline S120 degree 2 poles (-21.649, 24.1142) (-21.649, 24.1608) (-21.6642, 24.2495) (-21.6741, 24.2862) knots 0 0 0 1 2 2 2
  line L201 (-21.6741, 24.2862) -> (-21.5254, 24.2862)
  line L202 (-21.5173, 25.4) -> (-21.6831, 25.4)
  line L203 (-21.6831, 25.4) -> (-21.6831, 25.6599)
  line L204 (-21.6831, 25.6599) -> (-22.3264, 25.6599)
  line L205 (-22.3264, 25.6599) -> (-22.2037, 25.4341)
  line L206 (-22.2037, 25.4341) -> (-22.356, 25.3713)
  line L207 (-22.356, 25.3713) -> (-22.5236, 25.6957)
  line L208 (-22.5236, 25.6957) -> (-22.5236, 25.8552)
  line L209 (-22.5236, 25.8552) -> (-21.6831, 25.8552)
  line L210 (-21.6831, 25.8552) -> (-21.6831, 26.0792)
  line L211 (-21.6831, 26.0792) -> (-21.5173, 26.0792)
  line L212 (-21.5173, 26.0792) -> (-21.5173, 25.4)
  spline S121 degree 2 poles (-22.0218, 26.9986) (-21.8981, 26.9986) (-21.7037, 26.9439) (-21.5702, 26.8382) (-21.4994, 26.6867) (-21.4994, 26.5891) knots 0 0 0 1 2 3 4 4 4
  spline S122 degree 2 poles (-21.4994, 26.5891) (-21.4994, 26.5048) (-21.5576, 26.3633) (-21.6822, 26.2602) (-21.8766, 26.202) (-22.0128, 26.202) knots 0 0 0 1 2 3 4 4 4
  spline S123 degree 2 poles (-22.0128, 26.202) (-22.1356, 26.202) (-22.33, 26.2575) (-22.4635, 26.3624) (-22.5343, 26.5147) (-22.5343, 26.6124) knots 0 0 0 1 2 3 4 4 4
  spline S124 degree 2 poles (-22.5343, 26.6124) (-22.5343, 26.6966) (-22.4761, 26.8382) (-22.3524, 26.9403) (-22.158, 26.9986) (-22.0218, 26.9986) knots 0 0 0 1 2 3 4 4 4
  spline S125 degree 2 poles (-22.0182, 26.3937) (-22.0029, 26.3937) (-21.9761, 26.3937) (-21.9626, 26.3955) knots 0 0 0 1 2 2 2
  line L213 (-21.9626, 26.3955) -> (-22.2332, 26.7781)
  spline S126 degree 2 poles (-22.2332, 26.7781) (-22.3094, 26.7513) (-22.382, 26.6608) (-22.382, 26.5998) knots 0 0 0 1 2 2 2
  spline S127 degree 2 poles (-22.382, 26.5998) (-22.382, 26.5568) (-22.3381, 26.4815) (-22.2485, 26.426) (-22.1123, 26.3937) (-22.0182, 26.3937) knots 0 0 0 1 2 3 4 4 4
  spline S128 degree 2 poles (-22.0155, 26.8059) (-22.028, 26.8059) (-22.0549, 26.805) (-22.0675, 26.805) knots 0 0 0 1 2 2 2
  line L214 (-22.0675, 26.805) -> (-21.7978, 26.4242)
  spline S129 degree 2 poles (-21.7978, 26.4242) (-21.7243, 26.4493) (-21.6517, 26.5398) (-21.6517, 26.5998) knots 0 0 0 1 2 2 2
  spline S130 degree 2 poles (-21.6517, 26.5998) (-21.6517, 26.6437) (-21.6965, 26.7199) (-21.7861, 26.7755) (-21.9232, 26.8059) (-22.0155, 26.8059) knots 0 0 0 1 2 3 4 4 4
  spline S131 degree 2 poles (-22.0218, 27.8776) (-21.8981, 27.8776) (-21.7037, 27.8229) (-21.5702, 27.7172) (-21.4994, 27.5658) (-21.4994, 27.4681) knots 0 0 0 1 2 3 4 4 4
  spline S132 degree 2 poles (-21.4994, 27.4681) (-21.4994, 27.3839) (-21.5576, 27.2423) (-21.6822, 27.1393) (-21.8766, 27.081) (-22.0128, 27.081) knots 0 0 0 1 2 3 4 4 4
  spline S133 degree 2 poles (-22.0128, 27.081) (-22.1356, 27.081) (-22.33, 27.1366) (-22.4635, 27.2414) (-22.5343, 27.3937) (-22.5343, 27.4914) knots 0 0 0 1 2 3 4 4 4
  spline S134 degree 2 poles (-22.5343, 27.4914) (-22.5343, 27.5756) (-22.4761, 27.7172) (-22.3524, 27.8194) (-22.158, 27.8776) (-22.0218, 27.8776) knots 0 0 0 1 2 3 4 4 4
  spline S135 degree 2 poles (-22.0182, 27.2728) (-22.0029, 27.2728) (-21.9761, 27.2728) (-21.9626, 27.2746) knots 0 0 0 1 2 2 2
  line L215 (-21.9626, 27.2746) -> (-22.2332, 27.6572)
  spline S136 degree 2 poles (-22.2332, 27.6572) (-22.3094, 27.6303) (-22.382, 27.5398) (-22.382, 27.4789) knots 0 0 0 1 2 2 2
  spline S137 degree 2 poles (-22.382, 27.4789) (-22.382, 27.4358) (-22.3381, 27.3606) (-22.2485, 27.305) (-22.1123, 27.2728) (-22.0182, 27.2728) knots 0 0 0 1 2 3 4 4 4
  spline S138 degree 2 poles (-22.0155, 27.685) (-22.028, 27.685) (-22.0549, 27.6841) (-22.0675, 27.6841) knots 0 0 0 1 2 2 2
  line L216 (-22.0675, 27.6841) -> (-21.7978, 27.3032)
  spline S139 degree 2 poles (-21.7978, 27.3032) (-21.7243, 27.3283) (-21.6517, 27.4188) (-21.6517, 27.4789) knots 0 0 0 1 2 2 2
  spline S140 degree 2 poles (-21.6517, 27.4789) (-21.6517, 27.5228) (-21.6965, 27.5989) (-21.7861, 27.6545) (-21.9232, 27.685) (-22.0155, 27.685) knots 0 0 0 1 2 3 4 4 4
  spline S141 degree 2 poles (-22.0218, 28.7566) (-21.8981, 28.7566) (-21.7037, 28.702) (-21.5702, 28.5962) (-21.4994, 28.4448) (-21.4994, 28.3471) knots 0 0 0 1 2 3 4 4 4
  spline S142 degree 2 poles (-21.4994, 28.3471) (-21.4994, 28.2629) (-21.5576, 28.1213) (-21.6822, 28.0183) (-21.8766, 27.96) (-22.0128, 27.96) knots 0 0 0 1 2 3 4 4 4
  spline S143 degree 2 poles (-22.0128, 27.96) (-22.1356, 27.96) (-22.33, 28.0156) (-22.4635, 28.1204) (-22.5343, 28.2728) (-22.5343, 28.3704) knots 0 0 0 1 2 3 4 4 4
  spline S144 degree 2 poles (-22.5343, 28.3704) (-22.5343, 28.4547) (-22.4761, 28.5962) (-22.3524, 28.6984) (-22.158, 28.7566) (-22.0218, 28.7566) knots 0 0 0 1 2 3 4 4 4
  spline S145 degree 2 poles (-22.0182, 28.1518) (-22.0029, 28.1518) (-21.9761, 28.1518) (-21.9626, 28.1536) knots 0 0 0 1 2 2 2
  line L217 (-21.9626, 28.1536) -> (-22.2332, 28.5362)
  spline S146 degree 2 poles (-22.2332, 28.5362) (-22.3094, 28.5093) (-22.382, 28.4188) (-22.382, 28.3579) knots 0 0 0 1 2 2 2
  spline S147 degree 2 poles (-22.382, 28.3579) (-22.382, 28.3149) (-22.3381, 28.2396) (-22.2485, 28.1841) (-22.1123, 28.1518) (-22.0182, 28.1518) knots 0 0 0 1 2 3 4 4 4
  spline S148 degree 2 poles (-22.0155, 28.564) (-22.028, 28.564) (-22.0549, 28.5631) (-22.0675, 28.5631) knots 0 0 0 1 2 2 2
  line L218 (-22.0675, 28.5631) -> (-21.7978, 28.1823)
  spline S149 degree 2 poles (-21.7978, 28.1823) (-21.7243, 28.2074) (-21.6517, 28.2979) (-21.6517, 28.3579) knots 0 0 0 1 2 2 2
  spline S150 degree 2 poles (-21.6517, 28.3579) (-21.6517, 28.4018) (-21.6965, 28.478) (-21.7861, 28.5335) (-21.9232, 28.564) (-22.0155, 28.564) knots 0 0 0 1 2 3 4 4 4
  spline S151 degree 2 poles (-21.5567, 29.5819) (-21.5298, 29.5138) (-21.5038, 29.3866) (-21.5038, 29.3176) knots 0 0 0 1 2 2 2
  spline S152 degree 2 poles (-21.5038, 29.3176) (-21.5038, 29.2074) (-21.5675, 29.038) (-21.6929, 28.9224) (-21.8784, 28.8615) (-22.0021, 28.8615) knots 0 0 0 1 2 3 4 4 4
  spline S153 degree 2 poles (-22.0021, 28.8615) (-22.1284, 28.8615) (-22.3246, 28.9278) (-22.4599, 29.0496) (-22.5316, 29.2235) (-22.5316, 29.3319) knots 0 0 0 1 2 3 4 4 4
  spline S154 degree 2 poles (-22.5316, 29.3319) (-22.5316, 29.3669) (-22.528, 29.4287) (-22.52, 29.4878) (-22.5056, 29.5488) (-22.4949, 29.5819) knots 0 0 0 1 2 3 4 4 4
  line L219 (-22.4949, 29.5819) -> (-22.3085, 29.5819)
  spline S155 degree 2 poles (-22.3085, 29.5819) (-22.339, 29.5156) (-22.365, 29.3946) (-22.365, 29.3462) knots 0 0 0 1 2 2 2
  spline S156 degree 2 poles (-22.365, 29.3462) (-22.365, 29.2737) (-22.3139, 29.1706) (-22.2216, 29.1034) (-22.0935, 29.0729) (-22.0173, 29.0729) knots 0 0 0 1 2 3 4 4 4
  spline S157 degree 2 poles (-22.0173, 29.0729) (-21.9357, 29.0729) (-21.8085, 29.1043) (-21.7189, 29.1715) (-21.6723, 29.2764) (-21.6723, 29.348) knots 0 0 0 1 2 3 4 4 4
  spline S158 degree 2 poles (-21.6723, 29.348) (-21.6723, 29.374) (-21.6822, 29.4341) (-21.6983, 29.4959) (-21.7207, 29.5559) (-21.7323, 29.5819) knots 0 0 0 1 2 3 4 4 4
  line L220 (-21.7323, 29.5819) -> (-21.5567, 29.5819)
  spline S159 degree 2 poles (-2.0203, 7.4911) (-2.0006, 7.4391) (-1.9809, 7.3298) (-1.9809, 7.2716) knots 0 0 0 1 2 2 2
  spline S160 degree 2 poles (-1.9809, 7.2716) (-1.9809, 7.0897) (-2.178, 6.8926) (-2.368, 6.8926) knots 0 0 0 1 2 2 2
  spline S161 degree 2 poles (-2.368, 6.8926) (-2.4594, 6.8926) (-2.6072, 6.949) (-2.713, 7.0521) (-2.7703, 7.1945) (-2.7703, 7.2797) knots 0 0 0 1 2 3 4 4 4
  spline S162 degree 2 poles (-2.7703, 7.2797) (-2.7703, 7.3397) (-2.7533, 7.4436) (-2.7345, 7.4911) knots 0 0 0 1 2 2 2
  line L221 (-2.7345, 7.4911) -> (-2.6072, 7.4911)
  spline S163 degree 2 poles (-2.6072, 7.4911) (-2.6332, 7.4409) (-2.6574, 7.3379) (-2.6574, 7.2823) knots 0 0 0 1 2 2 2
  spline S164 degree 2 poles (-2.6574, 7.2823) (-2.6574, 7.2313) (-2.618, 7.1399) (-2.5445, 7.0709) (-2.4388, 7.0314) (-2.3725, 7.0314) knots 0 0 0 1 2 3 4 4 4
  spline S165 degree 2 poles (-2.3725, 7.0314) (-2.2336, 7.0314) (-2.0947, 7.1667) (-2.0947, 7.2877) knots 0 0 0 1 2 2 2
  spline S166 degree 2 poles (-2.0947, 7.2877) (-2.0947, 7.3415) (-2.1198, 7.4436) (-2.144, 7.4911) knots 0 0 0 1 2 2 2
  line L222 (-2.144, 7.4911) -> (-2.0203, 7.4911)
  line L223 (-1.9916, 8.3746) -> (-1.9916, 8.2411)
  line L224 (-1.9916, 8.2411) -> (-2.4827, 8.2411)
  spline S167 degree 2 poles (-2.4827, 8.2411) (-2.5714, 8.2411) (-2.6592, 8.1748) (-2.6592, 8.113) knots 0 0 0 1 2 2 2
  spline S168 degree 2 poles (-2.6592, 8.113) (-2.6592, 8.0861) (-2.6449, 8.0395) (-2.609, 7.9884) (-2.5472, 7.9293) (-2.5015, 7.8899) knots 0 0 0 1 2 3 4 4 4
  line L225 (-2.5015, 7.8899) -> (-1.9916, 7.8899)
  line L226 (-1.9916, 7.8899) -> (-1.9916, 7.7564)
  line L227 (-1.9916, 7.7564) -> (-3.0732, 7.7564)
  line L228 (-3.0732, 7.7564) -> (-3.0732, 7.8899)
  line L229 (-3.0732, 7.8899) -> (-2.7604, 7.8899)
  line L230 (-2.7604, 7.8899) -> (-2.6395, 7.8854)
  spline S169 degree 2 poles (-2.6395, 7.8854) (-2.6771, 7.9167) (-2.7282, 7.9768) (-2.7604, 8.0377) (-2.7739, 8.1004) (-2.7739, 8.1345) knots 0 0 0 1 2 3 4 4 4
  spline S170 degree 2 poles (-2.7739, 8.1345) (-2.7739, 8.2492) (-2.6341, 8.3746) (-2.4934, 8.3746) knots 0 0 0 1 2 2 2
  line L231 (-2.4934, 8.3746) -> (-1.9916, 8.3746)
  line L232 (-2.7596, 8.6497) -> (-2.7596, 8.7716)
  line L233 (-2.7596, 8.7716) -> (-2.618, 8.7752)
  spline S171 degree 2 poles (-2.618, 8.7752) (-2.7004, 8.8433) (-2.7739, 8.975) (-2.7739, 9.0431) knots 0 0 0 1 2 2 2
  spline S172 degree 2 poles (-2.7739, 9.0431) (-2.7739, 9.1623) (-2.6189, 9.285) (-2.4665, 9.2805) knots 0 0 0 1 2 2 2
  line L234 (-2.4665, 9.2805) -> (-2.4665, 9.1461)
  spline S173 degree 2 poles (-2.4665, 9.1461) (-2.5678, 9.1488) (-2.6592, 9.0852) (-2.6592, 9.0234) knots 0 0 0 1 2 2 2
  spline S174 degree 2 poles (-2.6592, 9.0234) (-2.6592, 8.9965) (-2.6404, 8.9427) (-2.5974, 8.8854) (-2.532, 8.8209) (-2.4845, 8.7841) knots 0 0 0 1 2 3 4 4 4
  line L235 (-2.4845, 8.7841) -> (-1.9916, 8.7841)
  line L236 (-1.9916, 8.7841) -> (-1.9916, 8.6497)
  line L237 (-1.9916, 8.6497) -> (-2.7596, 8.6497)
  spline S175 degree 2 poles (-2.6511, 10.0332) (-2.6242, 10.0547) (-2.5535, 10.078) (-2.5122, 10.078) knots 0 0 0 1 2 2 2
  spline S176 degree 2 poles (-2.5122, 10.078) (-2.4522, 10.078) (-2.3536, 10.0341) (-2.2837, 9.9553) (-2.2443, 9.8442) (-2.2443, 9.7779) knots 0 0 0 1 2 3 4 4 4
  spline S177 degree 2 poles (-2.2443, 9.7779) (-2.2443, 9.7295) (-2.2649, 9.6452) (-2.2802, 9.621) knots 0 0 0 1 2 2 2
  spline S178 degree 2 poles (-2.2802, 9.621) (-2.2587, 9.6058) (-2.221, 9.5861) (-2.1968, 9.5861) knots 0 0 0 1 2 2 2
  spline S179 degree 2 poles (-2.1968, 9.5861) (-2.1682, 9.5861) (-2.1296, 9.6417) (-2.1278, 9.6883) knots 0 0 0 1 2 2 2
  line L238 (-2.1278, 9.6883) -> (-2.1207, 9.8899)
  spline S180 degree 2 poles (-2.1207, 9.8899) (-2.1189, 9.9472) (-2.0929, 10.0449) (-2.0436, 10.1139) (-1.9719, 10.1533) (-1.9244, 10.1533) knots 0 0 0 1 2 3 4 4 4
  spline S181 degree 2 poles (-1.9244, 10.1533) (-1.8733, 10.1533) (-1.7811, 10.1085) (-1.7112, 10.0162) (-1.6699, 9.8737) (-1.6699, 9.7761) knots 0 0 0 1 2 3 4 4 4
  spline S182 degree 2 poles (-1.6699, 9.7761) (-1.6699, 9.6829) (-1.6995, 9.5521) (-1.7524, 9.4678) (-1.825, 9.4293) (-1.8689, 9.4293) knots 0 0 0 1 2 3 4 4 4
  spline S183 degree 2 poles (-1.8689, 9.4293) (-1.9253, 9.4293) (-2.0096, 9.4813) (-2.0481, 9.5359) knots 0 0 0 1 2 2 2
  spline S184 degree 2 poles (-2.0481, 9.5359) (-2.057, 9.5153) (-2.0848, 9.4866) (-2.118, 9.4678) (-2.1547, 9.4589) (-2.1726, 9.4589) knots 0 0 0 1 2 3 4 4 4
  spline S185 degree 2 poles (-2.1726, 9.4589) (-2.2219, 9.4589) (-2.3044, 9.5055) (-2.3411, 9.5377) knots 0 0 0 1 2 2 2
  spline S186 degree 2 poles (-2.3411, 9.5377) (-2.359, 9.5234) (-2.3931, 9.501) (-2.4316, 9.4848) (-2.4773, 9.4768) (-2.506, 9.4768) knots 0 0 0 1 2 3 4 4 4
  spline S187 degree 2 poles (-2.506, 9.4768) (-2.566, 9.4768) (-2.6646, 9.5207) (-2.7345, 9.5995) (-2.7739, 9.7098) (-2.7739, 9.777) knots 0 0 0 1 2 3 4 4 4
  spline S188 degree 2 poles (-2.7739, 9.777) (-2.7739, 9.8056) (-2.7658, 9.8576) (-2.7596, 9.8773) knots 0 0 0 1 2 2 2
  line L239 (-2.7596, 9.8773) -> (-2.7596, 10.156)
  line L240 (-2.7596, 10.156) -> (-2.6511, 10.156)
  line L241 (-2.6511, 10.156) -> (-2.6511, 10.0332)